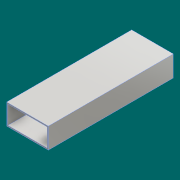
# Autodesk Inventor part: tube
Saved by Autodesk Inventor 2016 (Build 200138000, 138)
## iProperties
Created: 2016-07-19
Part Number: tube
Material: Aluminum 6061
Document SubType Name: Modeling
Designer: Jonathan
Density: 2.7 g/cm^3
Appearance: Aluminum - Flat
Author: Jonathan
Autodesk Inventor part; units mm, degrees
ref_plane "YZ Plane" through (0, 0, 0) normal (1, 0, 0) x (0, 1, 0)
ref_plane "XZ Plane" through (0, 0, 0) normal (0, 1, 0) x (-1, 0, 0)
ref_plane "XY Plane" through (0, 0, 0) normal (0, 0, 1) x (1, 0, 0)
sketch "Sketch1" plane through (0, 0, 0) normal (0, 1, 0) x (-1, 0, 0)
  line L0 (76.2, 25.4) -> (-76.2, 25.4)
  line L1 (-76.2, 25.4) -> (-76.2, -25.4)
  line L2 (-76.2, -25.4) -> (76.2, -25.4)
  line L3 (76.2, -25.4) -> (76.2, 25.4)
  line L4 (-73.025, 22.225) -> (73.025, 22.225)
  line L5 (73.025, 22.225) -> (73.025, -22.225)
  line L6 (73.025, -22.225) -> (-73.025, -22.225)
  line L7 (-73.025, -22.225) -> (-73.025, 22.225)
  point P0 (0, 0)
  point P1 (76.2, 0)
  point P2 (0, 25.4)
  dimension "d0" = 50.8
  dimension "d1" = 152.4
  dimension "d7" = 3.175
  constraints: 16 end point, 4 parallel, 2 midpoint, 2 perpendicular, 1 horizontal, 1 horizontal alignment, 1 vertical alignment, 3 other
  measures "d0" distance of L2.end L0.start
  measures "d1" distance of L1.end L2.end
  measures "d7" distance between parallel lines of L0 L4
extrude "Extrusion1" add sketch "Sketch1" along normal blind 304.8
equation "\"d0\" = tubeHeight"
equation "\"d1\" = tubeWidth"
equation "\"d7\" = tubeWallThickness"
equation "\"d4\" = tubeLength"
equation "\"nomTubeHeight\" = 50.8"
equation "\"nomTubeWidth\" = 152.4"
equation "\"tubeWallThickness\" = 3.175"
equation "\"nomTubeLength\" = 304.8"
equation "\"tubeWidth\" = 152.4"
equation "\"tubeHeight\" = 50.8"
equation "\"tubeLength\" = 304.8"
equation "\"plateOverhang\" = 6.35"
equation "\"moatWidth\" = 3.175"
equation "\"tubePlateClearance\" = 0.127"
equation "\"moatDepth\" = 3.175"
equation "\"blankCapThickness\" = 9.525"
equation "\"sensorCapThickness\" = 12.7"
equation "\"glassTubeDiameter\" = 12.7"
equation "\"glassTubeClearance\" = 0.19844"
equation "\"shortHoleSpacing\" = 21.59"
equation "\"longHoleSpacing\" = 30.48"
equation "\"fiberDiameter\" = 1"
equation "\"oRingID\" = 22.2504"
equation "\"oRingGrooveDepth\" = 1.2446"
equation "\"oRingGrooveWidth\" = 2.54"
equation "\"sensorHolderDiameter\" = 50.8"
equation "\"sensorHolderThickness\" = 12.7"
equation "\"fiberClearance\" = 0"
equation "\"glassTubeLength\" = 279.4"
equation "\"glassTubeID\" = 7.874"
equation "\"sensorBoardHoleSpacing\" = 19"
body "Solid1"
